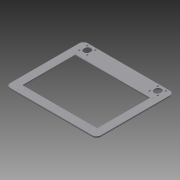
# Autodesk Inventor part: core xy plate
Saved by Autodesk Inventor 2014 SP1 (Build 180222100, 222)
## iProperties
Created: 2014-09-21
Part Number: core xy plate
Material: Generic
Document SubType Name: Modeling
Designer: Mon
Density: 1 g/cm^3
Appearance: Default
Author: Mon
Autodesk Inventor part; units mm, degrees
ref_plane "YZ Plane" through (0, 0, 0) normal (1, 0, 0) x (0, 1, 0)
ref_plane "XZ Plane" through (0, 0, 0) normal (0, 1, 0) x (-1, 0, 0)
ref_plane "XY Plane" through (0, 0, 0) normal (0, 0, 1) x (1, 0, 0)
sketch "Sketch1" plane through (0, 0, 0) normal (0, 1, 0) x (-1, 0, 0)
  line L0 (317.7202, 61.6798) -> (30.3202, 61.6798)
  line L1 (317.7202, 264.8798) -> (317.7202, 61.6798)
  line L2 (30.3202, 264.8798) -> (317.7202, 264.8798)
  line L3 (30.3202, 61.6798) -> (30.3202, 264.8798)
  arc A0 (0.0202, 15.9798) -> (16.0202, -0.0202) centre (16.0202, 15.9798) ccw
  line L4 (0.0202, 15.9798) -> (0.0202, 281.8798)
  arc A1 (16.0202, 297.8798) -> (0.0202, 281.8798) centre (16.0202, 281.8798) ccw
  line L5 (16.0202, 297.8798) -> (332.0202, 297.8798)
  arc A2 (348.0202, 281.8798) -> (332.0202, 297.8798) centre (332.0202, 281.8798) ccw
  line L6 (348.0202, 281.8798) -> (348.0202, 15.9798)
  arc A3 (332.0202, -0.0202) -> (348.0202, 15.9798) centre (332.0202, 15.9798) ccw
  line L7 (332.0202, -0.0202) -> (16.0202, -0.0202)
  arc A4 (21.2952, 6.4798) -> (25.0452, 6.4798) centre (23.1702, 6.4798) ccw
  line L8 (25.0452, 10.4798) -> (25.0452, 6.4798)
  arc A5 (25.0452, 10.4798) -> (21.2952, 10.4798) centre (23.1702, 10.4798) ccw
  line L9 (21.2952, 6.4798) -> (21.2952, 10.4798)
  arc A6 (52.2952, 6.4798) -> (56.0452, 6.4798) centre (54.1702, 6.4798) ccw
  line L10 (56.0452, 10.4798) -> (56.0452, 6.4798)
  arc A7 (56.0452, 10.4798) -> (52.2952, 10.4798) centre (54.1702, 10.4798) ccw
  line L11 (52.2952, 6.4798) -> (52.2952, 10.4798)
  arc A8 (21.2952, 37.4798) -> (25.0452, 37.4798) centre (23.1702, 37.4798) ccw
  line L12 (25.0452, 41.4798) -> (25.0452, 37.4798)
  arc A9 (25.0452, 41.4798) -> (21.2952, 41.4798) centre (23.1702, 41.4798) ccw
  line L13 (21.2952, 37.4798) -> (21.2952, 41.4798)
  arc A10 (52.2952, 37.4798) -> (56.0452, 37.4798) centre (54.1702, 37.4798) ccw
  line L14 (56.0452, 41.4798) -> (56.0452, 37.4798)
  arc A11 (56.0452, 41.4798) -> (52.2952, 41.4798) centre (54.1702, 41.4798) ccw
  line L15 (52.2952, 37.4798) -> (52.2952, 41.4798)
  arc A12 (26.6702, 21.9798) -> (50.6702, 21.9798) centre (38.6702, 21.9798) ccw
  line L16 (50.6702, 25.9798) -> (50.6702, 21.9798)
  arc A13 (50.6702, 25.9798) -> (26.6702, 25.9798) centre (38.6702, 25.9798) ccw
  line L17 (26.6702, 21.9798) -> (26.6702, 25.9798)
  arc A14 (291.9952, 6.4798) -> (295.7452, 6.4798) centre (293.8702, 6.4798) ccw
  line L18 (295.7452, 10.4798) -> (295.7452, 6.4798)
  arc A15 (295.7452, 10.4798) -> (291.9952, 10.4798) centre (293.8702, 10.4798) ccw
  line L19 (291.9952, 6.4798) -> (291.9952, 10.4798)
  arc A16 (322.9952, 6.4798) -> (326.7452, 6.4798) centre (324.8702, 6.4798) ccw
  line L20 (326.7452, 10.4798) -> (326.7452, 6.4798)
  line L21 (322.9952, 6.4798) -> (322.9952, 10.4798)
  arc A17 (322.9952, 37.4798) -> (326.7452, 37.4798) centre (324.8702, 37.4798) ccw
  line L22 (326.7452, 41.4798) -> (326.7452, 37.4798)
  arc A18 (326.7452, 41.4798) -> (322.9952, 41.4798) centre (324.8702, 41.4798) ccw
  line L23 (322.9952, 37.4798) -> (322.9952, 41.4798)
  arc A19 (291.9952, 37.4798) -> (295.7452, 37.4798) centre (293.8702, 37.4798) ccw
  line L24 (295.7452, 41.4798) -> (295.7452, 37.4798)
  arc A20 (295.7452, 41.4798) -> (291.9952, 41.4798) centre (293.8702, 41.4798) ccw
  line L25 (291.9952, 37.4798) -> (291.9952, 41.4798)
  arc A21 (297.3702, 21.9798) -> (321.3702, 21.9798) centre (309.3702, 21.9798) ccw
  line L26 (321.3702, 25.9798) -> (321.3702, 21.9798)
  arc A22 (321.3702, 25.9798) -> (297.3702, 25.9798) centre (309.3702, 25.9798) ccw
  line L27 (297.3702, 21.9798) -> (297.3702, 25.9798)
  circle A23 centre (50.2702, 272.8798) radius 1
  circle A24 centre (38.6702, 287.8798) radius 1
  circle A25 centre (309.3702, 287.8798) radius 1
  circle A26 centre (297.7702, 272.8798) radius 1
  circle A27 centre (25.9077, 270.3798) radius 1
  circle A28 centre (66.9077, 270.3798) radius 1
  circle A29 centre (174.0202, 270.3798) radius 1
  circle A30 centre (281.1327, 270.3798) radius 1
  circle A31 centre (322.1327, 270.3798) radius 1
  circle A32 centre (322.1327, 56.1798) radius 1
  circle A33 centre (281.1327, 56.1798) radius 1
  circle A34 centre (174.0202, 56.1798) radius 1
  circle A35 centre (66.9077, 56.1798) radius 1
  circle A36 centre (25.9077, 56.1798) radius 1
  arc A37 (326.7452, 10.4798) -> (322.9952, 10.4798) centre (324.8702, 10.4798) ccw
  point P0 (0, 0)
  constraints: 56 end point, 48 point on circle, 38 centre point
extrude "Extrusion1" add sketch "Sketch1" along normal blind 4.7625
body "Solid1"
